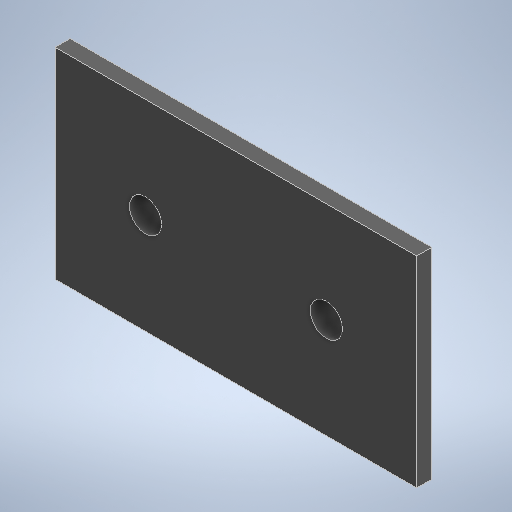
# Autodesk Inventor part: belt_fix
Saved by Autodesk Inventor 2026.1 (Build 301233020, 233B)
## iProperties
Created: 2026-02-04
Part Number: belt_fix
Material: 一般
Document SubType Name: Modeling
Designer: hibik
Density: 1 g/cm^3
Appearance: 既定
Author: hibik
Autodesk Inventor part; units mm, degrees
ref_plane "YZ Plane" through (0, 0, 0) normal (1, 0, 0) x (0, 1, 0)
ref_plane "XZ Plane" through (0, 0, 0) normal (0, 1, 0) x (-1, 0, 0)
ref_plane "XY Plane" through (0, 0, 0) normal (0, 0, 1) x (1, 0, 0)
sketch "スケッチ1" plane through (0, 0, 0) normal (0, 0, 1) x (1, 0, 0)
  line L0 (-18, 10) -> (18, 10)
  line L1 (18, 10) -> (18, -10)
  line L2 (18, -10) -> (-18, -10)
  line L3 (-18, -10) -> (-18, 10)
  point P0 (0, 0)
  point P1 (0, 10)
  point P2 (-18, 0)
  dimension "d0" = 36
  dimension "d1" = 20
  constraints: 8 end point, 2 midpoint, 2 parallel, 1 horizontal, 1 horizontal alignment, 1 perpendicular, 1 vertical alignment
  measures "d0" distance of L0.start L0.end
  measures "d1" distance of L0.end L1.end
extrude "押し出し1" add sketch "スケッチ1" along normal blind 1.5
sketch "スケッチ2" plane through (0, 0, 0) normal (0, 0, -1) x (-1, 0, 0)
  circle A0 centre (-9, 0) radius 2.75
  circle A1 centre (9, 0) radius 2.75
  line L0 (0, -50.45) -> (0, 52.45) projected
  line L1 (-18, 10) -> (18, 10) projected
  point P0 (0, 0)
  dimension "d4" = 5.5
  dimension "d5" = 9
  dimension "d6" = 10
  constraints: 2 centre point, 1 other
  measures "d4" diameter of A0
  measures "d5" distance from line of L0 A0.centre
  measures "d6" distance from line of L1 A0.centre
extrude "押し出し2" add sketch "スケッチ2" along normal blind 2.5
sketch "スケッチ3" plane through (-9, 0, -2.5) normal (0, 0, -1) x (-1, 0, 0)
  circle A0 centre (0, 0) radius 2.75 construction
  circle A1 centre (-18, 0) radius 2.75 construction
  circle A2 centre (0, 0) radius 1.6
  circle A3 centre (-18, 0) radius 1.6
  line L0 (-9, -85.52) -> (-9, 25.92) projected
  point P0 (-9, 0)
  dimension "d16" = 3.2
  dimension "d17" = 3.2
  constraints: 2 centre point, 2 coincident
  measures "d16" diameter of A2
  measures "d17" diameter of A3
extrude "押し出し3" cut sketch "スケッチ3" against normal through all
